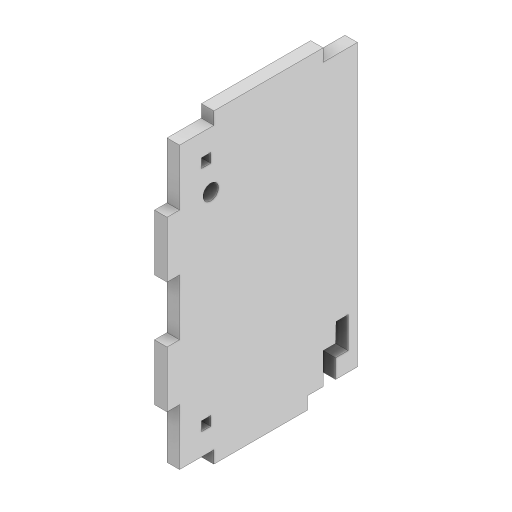
# Autodesk Inventor part: Side
Saved by Autodesk Inventor 2023.3 (Build 273359000, 359)
## iProperties
Created: 2024-06-25
Part Number: Side
Material: Generic
Document SubType Name: Modeling
Designer: David Zindović
Density: 1 g/cm^3
Appearance: Default
Author: David Zindović
Autodesk Inventor part; units mm, degrees
ref_plane "YZ Plane" through (0, 0, 0) normal (1, 0, 0) x (0, 1, 0)
ref_plane "XZ Plane" through (0, 0, 0) normal (0, 1, 0) x (-1, 0, 0)
ref_plane "XY Plane" through (0, 0, 0) normal (0, 0, 1) x (1, 0, 0)
sketch "Sketch1" plane through (0, 0, 0) normal (1, 0, 0) x (0, 1, 0)
  line L0 (-45, 21) -> (45, 21)
  line L1 (45, 21) -> (45, -21)
  line L2 (-27, 21) -> (-9, 21)
  line L3 (-9, 21) -> (-9, 25)
  line L4 (-9, 25) -> (-27, 25)
  line L5 (-27, 25) -> (-27, 21)
  line L6 (9, 21) -> (27, 21)
  line L7 (27, 21) -> (27, 25)
  line L8 (27, 25) -> (9, 25)
  line L9 (9, 25) -> (9, 21)
  line L10 (-45, 10) -> (-49, 10)
  line L11 (-49, 10) -> (-49, -10)
  line L12 (-49, -10) -> (-45, -10) construction
  line L13 (-45, -10) -> (-45, 10)
  line L14 (45, 10) -> (49, 10)
  line L15 (49, 10) -> (49, -10)
  line L16 (49, -10) -> (45, -10) construction
  line L17 (45, -10) -> (45, 10)
  line L18 (-45, -21) -> (-45, 21)
  line L19 (45, 21) -> (45, -36)
  line L20 (45, -36) -> (-45, -36)
  line L21 (-45, -36) -> (-45, 21)
  line L22 (45, 10) -> (49, 10)
  line L23 (49, 10) -> (49, -20)
  line L24 (49, -20) -> (45, -20)
  line L25 (45, -20) -> (45, 10)
  line L26 (-45, 10) -> (-49, 10)
  line L27 (-49, 10) -> (-49, -20)
  line L28 (-49, -20) -> (-45, -20) construction
  line L29 (-45, -20) -> (-45, 10)
  line L30 (-18, -36) -> (-22, -36)
  line L31 (-45, -29) -> (-39, -29)
  line L32 (-39, -29) -> (-39, -25)
  line L33 (-39, -25) -> (-45, -25)
  line L34 (-45, -25) -> (-45, -29)
  line L35 (-39, -25) -> (-35, -25)
  line L36 (-35, -25) -> (-35, -33)
  line L37 (-35, -33) -> (-39, -33)
  line L38 (-39, -33) -> (-39, -25)
  line L39 (-35, -33) -> (-29, -33)
  line L40 (-29, -33) -> (-29, -29)
  line L41 (-29, -29) -> (-35, -29)
  line L42 (-35, -29) -> (-35, -33)
  line L43 (-29, -29) -> (-29, -29.15)
  line L44 (-29, -29.15) -> (-35, -29)
  line L45 (49, -20) -> (45, -20) construction
  line L46 (45, -20) -> (45, -25)
  line L47 (45, -25) -> (49, -25)
  line L48 (49, -25) -> (49, -20)
  line L49 (-45, -20) -> (-49, -20) construction
  line L50 (-49, -20) -> (-49, -25)
  line L51 (-49, -25) -> (-45, -25)
  line L52 (-45, -25) -> (-45, -20)
  line L53 (-45, -25) -> (-49, -25)
  line L54 (-49, -25) -> (-49, -20)
  line L55 (-49, -20) -> (-45, -20)
  line L56 (-45, -20) -> (-45, -25)
  point P0 (0, 0)
  point P1 (0, 21)
  point P2 (45, 0)
  point P3 (-9, 23)
  point P4 (9, 23)
  point P5 (49, 0)
  point P6 (45, -10)
  point P7 (27, 21)
  point P8 (-45, 10)
  point P9 (-45, -20)
  point P10 (-45, -20)
  point P11 (-35, -29)
  point P12 (-32, -33)
  point P13 (-32, -29)
  point P14 (-47, 10)
  point P15 (47, 10)
  dimension "d9" = 18
  dimension "d10" = 18
  dimension "d11" = 18
  dimension "d12" = 18
  dimension "d13" = 4
  dimension "d17" = 20
  dimension "d19" = 20
  dimension "d20" = 4
  dimension "d21" = 4
  dimension "d40" = 42
  dimension "d41" = 57
  dimension "d42" = 30
  dimension "d43" = 30
  dimension "d47" = 6
  dimension "d48" = 4
  dimension "d49" = 7
  dimension "d50" = 4
  dimension "d51" = 8
  dimension "d52" = 6
  dimension "d55" = 4
  dimension "d56" = 0.15
  constraints: 114 end point, 20 parallel, 13 horizontal, 11 perpendicular, 9 midpoint, 6 point on line, 3 horizontal alignment, 2 vertical, 2 vertical alignment
  measures "d9" distance of L3.end L4.end
  measures "d10" horizontal distance of L0.start L4.end
  measures "d11" distance of L7.end L8.end
  measures "d12" distance of point (-9, 23) point (9, 23)
  measures "d13" distance of L6.end L7.end
  measures "d17" distance of L10.end L11.end
  measures "d19" distance of L14.end L15.end
  measures "d20" distance of L10.start L10.end
  measures "d21" distance of L14.start L14.end
  measures "d40" distance of L0.end L1.end
  measures "d41" distance of L0.end L19.end
  measures "d42" distance of L22.end L23.end
  measures "d43" distance of L27.end L26.end
  measures "d47" distance of L33.end L32.end
  measures "d48" distance of L32.end L31.end
  measures "d49" distance between parallel lines of L20 L31
  measures "d50" distance of L36.end L37.end
  measures "d51" distance of L35.end L36.end
  measures "d52" distance of L41.end L40.end
  measures "d55" distance of point (-32, -33) point (-32, -29)
  measures "d56" distance of L40.end L43.end
extrude "Extrusion1" add sketch "Sketch1" along normal mid plane 4 contours L0 L1 L19 L20 L21 L31 L38 L37 L39 L40 L41 L36 L35 L33 L18 L13 | L5 L4 L3 L0 | L13 L18 L55 L27 L11 L10 | L9 L8 L7 L0 | L14 L15 L23 L24 L1 | L24 L48 L47 L19 L1 | L41 L40 L44
sketch "Sketch2" plane through (2, 0, 0) normal (1, 0, 0) x (0, 0, -1)
  circle A0 centre (-11, 27) radius 2.5
  line L0 (14, -45) -> (14, -25) projected
  line L1 (-10, 45) -> (-21, 45) projected
  line L2 (6.5, -45) -> (14, -45) projected
  circle A1 centre (-12.5, -36.5) radius 1.55 construction
  line L3 (-21, -45) -> (-10, -45) projected
  line L4 (-21, 9) -> (-21, 27) projected
  line L5 (0, 0) -> (-4.5, 0)
  circle A2 centre (-12.5, 36.5) radius 1.55 construction
  line L6 (-14, 38) -> (-11, 38)
  line L7 (-11, 38) -> (-11, 35)
  line L8 (-11, 35) -> (-14, 35)
  line L9 (-14, 35) -> (-14, 38)
  line L10 (-14, -35) -> (-11, -35)
  line L11 (-11, -35) -> (-11, -38)
  line L12 (-11, -38) -> (-14, -38)
  line L13 (-14, -38) -> (-14, -35)
  line L14 (-25, -9) -> (-25, -27) projected
  line L15 (-10, -49) -> (20, -49) projected
  point P0 (21, 45)
  point P1 (10, 45)
  point P2 (-15.5, 45)
  point P3 (10.25, -45)
  point P4 (-15.5, -45)
  point P5 (-21, -27)
  point P6 (-12.5, 38)
  point P7 (-14, 36.5)
  point P8 (-12.5, -35)
  point P9 (-11, -36.5)
  point P10 (16.5, -49)
  point P11 (25, -49)
  dimension "d24" = 5
  dimension "d25" = 25
  dimension "d26" = 18
  dimension "d33" = 3.1
  dimension "d36" = 3
  dimension "d37" = 3
  dimension "d38" = 3
  dimension "d53" = 11
  dimension "d54" = 11
  constraints: 18 end point, 7 midpoint, 4 parallel, 3 centre point, 3 horizontal, 2 horizontal alignment, 2 perpendicular, 2 vertical alignment, 1 symmetric about line, 1 other
  measures "d24" diameter of A0
  measures "d25" distance from line of L0 A0.centre
  measures "d26" vertical distance of point (-15.5, 45) A0.centre
  measures "d33" diameter of A1
  measures "d36" distance of L7.end L8.end
  measures "d37" distance of L6.end L7.end
  measures "d38" distance of L11.end L12.end
  measures "d53" distance between parallel lines of L14 L13
  measures "d54" distance between parallel lines of L15 L12
extrude "Extrusion2" cut sketch "Sketch2" against normal up to surface (4 mm away)
equation "\"d9\" = 0.2 * d3"
equation "\"d10\" = d9"
equation "\"d11\" = d9"
equation "\"d12\" = d11"
equation "\"d17\" = d19"
equation "\"d20\" = d13"
equation "\"d21\" = d13"
equation "\"d54\" = d53"
equation "\"d3\" = 90"
body "Solid1"
